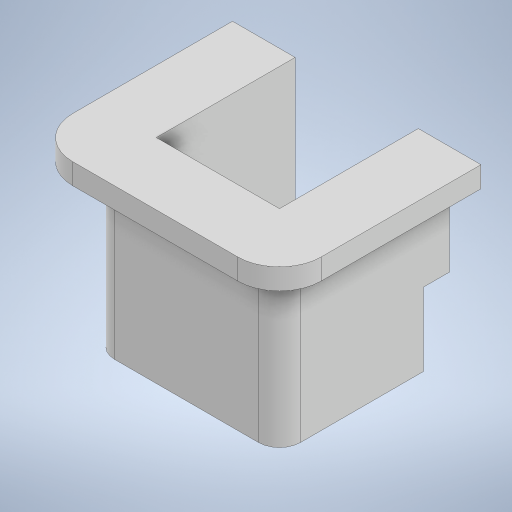
# Autodesk Inventor part: PIeza Conector USB
Saved by Autodesk Inventor 2024 (Build 280153000, 153)
## iProperties
Created: 2023-06-25
Part Number: PIeza Conector USB
Material: Genérico
Document SubType Name: Modeling
Designer: sergi
Density: 1 g/cm^3
Appearance: Valor por defecto
Author: sergi
Autodesk Inventor part; units mm, degrees
ref_plane "YZ Plane" through (0, 0, 0) normal (1, 0, 0) x (0, 1, 0)
ref_plane "XZ Plane" through (0, 0, 0) normal (0, 1, 0) x (-1, 0, 0)
ref_plane "XY Plane" through (0, 0, 0) normal (0, 0, 1) x (1, 0, 0)
sketch "Boceto1" plane through (0, 0, 0) normal (0, 1, 0) x (-1, 0, 0)
  line L0 (-2.95, -6.65) -> (2.95, -6.65)
  line L1 (2.95, -6.65) -> (2.95, 6.65)
  line L2 (2.95, 6.65) -> (-2.95, 6.65)
  line L3 (-2.95, 6.65) -> (-2.95, -6.65)
  line L4 (-2.95, -6.65) -> (2.95, 6.65) construction
  line L5 (2.95, -6.65) -> (-2.95, 6.65) construction
  line L6 (4.45, 8.15) -> (4.45, -8.15)
  line L7 (4.45, -8.15) -> (-4.45, -8.15)
  line L8 (-4.45, -8.15) -> (-4.45, 8.15)
  line L9 (-4.45, 8.15) -> (4.45, 8.15)
  point P0 (0, 0)
  dimension "d0" = 5.9
  dimension "d1" = 13.3
  dimension "d2" = 1.5
  constraints: 20 end point, 4 parallel, 2 midpoint, 2 perpendicular, 1 horizontal, 3 other
  measures "d0" distance of L2.end L1.end
  measures "d1" distance of L1.end L0.end
  measures "d2" distance between parallel lines of L1 L6
extrude "Extrusión1" add sketch "Boceto1" along normal blind 8.7
sketch "Boceto2" plane through (0, 8.7, 0) normal (0, 1, 0) x (1, 0, 0)
  line L0 (4.45, -8.15) -> (4.45, 8.15) projected
  line L1 (4.45, 8.15) -> (-4.45, 8.15) projected
  line L2 (-4.45, 8.15) -> (-4.45, -8.15) projected
  line L3 (-4.45, -8.15) -> (4.45, -8.15) projected
  line L4 (2.95, 6.65) -> (2.95, -6.65) projected
  line L5 (2.95, -6.65) -> (-2.95, -6.65) projected
  line L6 (-2.95, -6.65) -> (-2.95, 6.65) projected
  line L7 (-2.95, 6.65) -> (2.95, 6.65) projected
  line L8 (-5.95, -9.65) -> (-5.95, 9.65)
  line L9 (-5.95, 9.65) -> (5.95, 9.65)
  line L10 (5.95, 9.65) -> (5.95, -9.65)
  line L11 (5.95, -9.65) -> (-5.95, -9.65)
  point P0 (0, 0)
  dimension "d5" = 1.5
  constraints: 8 end point, 3 other
  measures "d5" distance between parallel lines of L2 L8
extrude "Extrusión2" add sketch "Boceto2" against normal blind 1 contours L8 L9 L10 L11
fillet "Empalme1" radius 2 4 edges at (5.95, 8.2, 9.65) (-5.95, 8.2, 9.65) (5.95, 8.2, -9.65) (-5.95, 8.2, -9.65)
fillet "Empalme2" radius 1 4 edges at (4.45, 3.85, 8.15) (-4.45, 3.85, 8.15) (4.45, 3.85, -8.15) (-4.45, 3.85, -8.15)
sketch "Boceto3" plane through (0, 0, 0) normal (0, -1, 0) x (1, 0, 0)
  line L0 (0, 0) -> (0, -1.25)
  line L1 (0, -1.25) -> (4.45, -1.25)
  line L2 (4.45, 7.15) -> (4.45, -7.15) projected
  line L3 (0, 0) -> (0, 1.25)
  line L4 (0, 1.25) -> (4.45, 1.25)
  dimension "d10" = 1.25
  dimension "d11" = 1.25
  constraints: 8 end point, 3 point on line, 2 perpendicular, 1 vertical
  measures "d10" distance of L0.start L0.end
  measures "d11" distance of L0.start L3.end
extrude "Extrusión3" cut sketch "Boceto3" against normal blind 3.5
split "Dividir1" plane through (0, 0, 0) removes the side toward (0, 0, -1)
